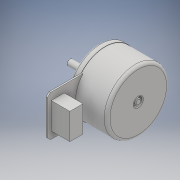
# Autodesk Inventor part: Brushless_70W
Saved by Autodesk Inventor 2017 (Build 210142000, 142)
## iProperties
Part Number: Brushless_70W
Material: Générique
Document SubType Name: Modeling
Designer: Darren
Density: 1 g/cm^3
Appearance: Par défaut
Author: Darren
Autodesk Inventor part; units mm, degrees
ref_plane "YZ Plane" through (0, 0, 0) normal (1, 0, 0) x (0, 1, 0)
ref_plane "XZ Plane" through (0, 0, 0) normal (0, 1, 0) x (-1, 0, 0)
ref_plane "XY Plane" through (0, 0, 0) normal (0, 0, 1) x (1, 0, 0)
sketch "Esquisse1" plane through (0, 0, 0) normal (0, 0, 1) x (1, 0, 0)
  line L0 (-56.76, 0) -> (9.46, 0) construction
  line L1 (0, -4.32) -> (0, 25.92) construction
  line L2 (-2, 0) -> (-26.7, 0)
  line L3 (-26.7, 0) -> (-26.7, 21.4)
  line L4 (-22.7, 21.4) -> (0, 21.4)
  line L5 (0, 21.4) -> (0, 3)
  line L6 (-26.7, 0) -> (-29.9, 0)
  line L7 (-29.9, 0) -> (-29.9, 6)
  line L8 (-29.9, 6) -> (-26.7, 6)
  line L9 (-26.7, 6) -> (-26.7, 0)
  line L10 (-29.9, 0) -> (-47.3, 0)
  line L11 (-47.3, 0) -> (-47.3, 2)
  line L12 (-47.3, 2) -> (-29.9, 2)
  line L13 (-29.9, 2) -> (-29.9, 0)
  line L14 (-26.7, 0) -> (-22.7, 0)
  line L15 (-22.7, 21.4) -> (-22.7, 21.6)
  line L16 (-22.7, 21.6) -> (-26.7, 21.6)
  line L17 (-26.7, 21.6) -> (-26.7, 0)
  line L18 (-2, 0) -> (-2, 3)
  line L19 (-2, 3) -> (0, 3)
  point P0 (0, 0)
  dimension "d2" = 3.2
  dimension "d3" = 6
  dimension "d4" = 17.4
  dimension "d5" = 2
  dimension "d17" = 0.2
  dimension "d18" = 4
  dimension "d47" = 2
  dimension "d48" = 3
  dimension "d49" = 21.4
  dimension "d50" = 26.7
  constraints: 36 end point, 8 parallel, 4 horizontal, 4 perpendicular, 2 collinear
  measures "d2" distance of L7.end L8.end
  measures "d3" distance of L6.end L7.end
  measures "d4" distance of L11.end L12.end
  measures "d5" distance of L10.end L11.end
  measures "d17" distance between parallel lines of L4 L16
  measures "d18" distance between parallel lines of L3 L15
  measures "d47" distance between parallel lines of L1 L18
  measures "d48" distance between parallel lines of L0 L19
  measures "d49" distance between parallel lines of L2 L4
  measures "d50" distance between parallel lines of L5 L3
revolve "Révolution1" add sketch "Esquisse1" angle 360 about axis through (-10, 0, 0) along (1, 0, 0)
sketch "Esquisse3" plane through (-26.7, 0, 0) normal (-1, 0, 0) x (0, 0, 1)
  circle A0 centre (0, 0) radius 21.6 construction
  circle A1 centre (0, 0) radius 6 construction
  line L0 (0, -30.24) -> (0, 30.24) construction
  circle A2 centre (0, 0) radius 2 construction
  circle A3 centre (0, 0) radius 11 construction
  circle A4 centre (0, 11) radius 1.5
  circle A5 centre (-9.5263, -5.5) radius 1.5
  circle A6 centre (9.5263, -5.5) radius 1.5
  line L1 (0, 0) -> (0, 11) construction
  line L2 (0, 0) -> (-9.5263, -5.5) construction
  circle A7 centre (0, 0) radius 3 construction
  line L3 (0, 0) -> (9.5263, -5.5) construction
  dimension "d20" = 22
  dimension "d21" = 3
  dimension "d24" = 360
  constraints: 6 end point, 3 centre point, 1 coincident, 1 collinear, 1 point on line, 1 vertical alignment, 9 other
  measures "d21" diameter of A4
extrude "Extrusion1" cut sketch "Esquisse3" against normal blind 3.9
sketch "Esquisse4" plane through (-22.7, 0, 0) normal (1, 0, 0) x (0, 0, -1)
  circle A0 centre (0, 0) radius 21.4 construction
  line L0 (0, -52.92) -> (0, 34.02) construction
  line L1 (30.24, 0) -> (-30.24, 0) construction
  line L2 (-14, 0) -> (14, 0)
  line L3 (14, 0) -> (14, -38.5)
  line L4 (12, -40.5) -> (-12, -40.5)
  line L5 (-14, -38.5) -> (-14, 0)
  line L6 (-14, -38.5) -> (-12, -40.5)
  line L7 (12, -40.5) -> (14, -38.5)
  circle A1 centre (0, 0) radius 21.6 construction
  point P0 (14, -40.5)
  point P1 (-14, -40.5)
  dimension "d28" = 28
  dimension "d29" = 40.5
  dimension "d30" = 14
  dimension "d31" = 2
  dimension "d32" = 2
  dimension "d33" = 2
  dimension "d34" = 2
  constraints: 12 end point, 5 point on line, 2 parallel, 1 horizontal, 1 perpendicular
  measures "d28" distance of point (14, -40.5) point (-14, -40.5)
  measures "d29" distance of L2.end point (14, -40.5)
  measures "d30" distance between parallel lines of L0 L5
  measures "d31" distance of L5.start point (-14, -40.5)
  measures "d32" distance of L4.end point (-14, -40.5)
  measures "d33" distance of L4.start point (14, -40.5)
  measures "d34" distance of L3.end point (14, -40.5)
extrude "Extrusion2" add sketch "Esquisse4" along normal blind 1
sketch "Esquisse5" plane through (-21.7, 0, 0) normal (1, 0, 0) x (0, 0, -1)
  line L0 (0, -52.92) -> (0, 34.02) construction
  line L1 (30.24, 0) -> (-30.24, 0) construction
  arc A0 (-14, -16.1852) -> (14, -16.1852) centre (0, 0) ccw construction
  line L2 (-14, -16.1852) -> (-14, -38.5) construction
  line L3 (-14, -38.5) -> (-12, -40.5) construction
  line L4 (-12, -40.5) -> (12, -40.5) construction
  line L5 (12, -40.5) -> (14, -38.5) construction
  line L6 (14, -38.5) -> (14, -16.1852) construction
  line L7 (-9, -29) -> (9, -29)
  line L8 (9, -29) -> (9, -38)
  line L9 (9, -38) -> (-9, -38)
  line L10 (-9, -38) -> (-9, -29)
  dimension "d37" = 18
  dimension "d38" = 9
  dimension "d39" = 9
  dimension "d40" = 2.5
  constraints: 8 end point, 2 parallel, 1 horizontal, 1 perpendicular
  measures "d37" distance of L8.end L9.end
  measures "d38" distance of L7.end L8.end
  measures "d39" distance between parallel lines of L0 L10
  measures "d40" distance between parallel lines of L4 L9
extrude "Extrusion3" add sketch "Esquisse5" along normal blind 12.8
sketch "Esquisse6" plane through (-2, 0, 0) normal (1, 0, 0) x (0, 0, -1)
  circle A0 centre (0, 0) radius 1.5 construction
  circle A1 centre (0, 0) radius 2 construction
  circle A2 centre (0, 0) radius 2
  dimension "d51" = 4
  constraints: 1 centre point, 1 coincident
  measures "d51" diameter of A2
extrude "Extrusion4" add sketch "Esquisse6" along normal blind 2
fillet "Congé2" radius 0.5 4 edges at (0, 0, 2) (0, -3, 0) (-29.9, -6, 0) (-47.3, -2, 0)
fillet "Congé2" radius 1 1 edges at (-26.7, -21.6, 0)
fillet "Congé2" radius 2 1 edges at (0, -21.4, 0)
equation "\"d32\" = d31"
equation "\"d33\" = d31"
equation "\"d34\" = d33"
